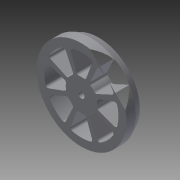
# Autodesk Inventor part: Colossus_7kW_Rotor
Saved by Autodesk Inventor 2014 (Build 180170000, 170)
## iProperties
Created: 2014-11-23
Part Number: Colossus_7kW_Rotor
Material: Générique
Document SubType Name: Modeling
Designer: Yann
Density: 1 g/cm^3
Appearance: Par défaut
Author: Yann
Autodesk Inventor part; units mm, degrees
ref_plane "YZ Plane" through (0, 0, 0) normal (1, 0, 0) x (0, 1, 0)
ref_plane "XZ Plane" through (0, 0, 0) normal (0, 1, 0) x (-1, 0, 0)
ref_plane "XY Plane" through (0, 0, 0) normal (0, 0, 1) x (1, 0, 0)
sketch "Esquisse1" plane through (0, 0, 0) normal (0, 1, 0) x (-1, 0, 0)
  arc A0 (26.7424, 50.7333) -> (-26.7424, 50.7333) centre (0, 0) ccw
  circle A1 centre (0, 0) radius 57.35
  line L0 (0, -80.29) -> (0, 80.29) construction
  line L1 (-80.29, 0) -> (80.29, 0) construction
  circle A2 centre (0, 0) radius 4
  line L2 (-6.2691, 21.7137) -> (-13.6461, 41.982)
  line L3 (13.6461, 41.982) -> (6.2691, 21.7137)
  arc A3 (11.5595, 45.9173) -> (-11.5595, 45.9173) centre (0, 0) ccw
  arc A4 (-11.5595, 45.9173) -> (-13.6461, 41.982) centre (-10.8271, 43.0081) ccw
  arc A5 (13.6461, 41.982) -> (11.5595, 45.9173) centre (10.8271, 43.0081) ccw
  circle A6 centre (0, 0) radius 16 construction
  circle A7 centre (0, 0) radius 57.35 construction
  arc A8 (3, 19.7737) -> (-3, 19.7737) centre (0, 0) ccw
  arc A9 (-6.2691, 21.7137) -> (-3, 19.7737) centre (-3.45, 22.7398) ccw
  arc A10 (3, 19.7737) -> (6.2691, 21.7137) centre (3.45, 22.7398) ccw
  line L4 (-19.7868, 10.921) -> (-39.3351, 20.0365)
  line L5 (-20.0365, 39.3351) -> (-10.921, 19.7868)
  arc A11 (-24.2947, 40.6422) -> (-40.6422, 24.2947) centre (0, 0) ccw
  arc A12 (-40.6422, 24.2947) -> (-39.3351, 20.0365) centre (-38.0672, 22.7554) ccw
  arc A13 (-20.0365, 39.3351) -> (-24.2947, 40.6422) centre (-22.7554, 38.0672) ccw
  arc A14 (-11.8608, 16.1035) -> (-16.1035, 11.8608) centre (0, 0) ccw
  arc A15 (-19.7868, 10.921) -> (-16.1035, 11.8608) centre (-18.519, 13.6399) ccw
  arc A16 (-11.8608, 16.1035) -> (-10.921, 19.7868) centre (-13.6399, 18.519) ccw
  line L6 (-21.7137, -6.2691) -> (-41.982, -13.6461)
  line L7 (-41.982, 13.6461) -> (-21.7137, 6.2691)
  arc A17 (-45.9173, 11.5595) -> (-45.9173, -11.5595) centre (0, 0) ccw
  arc A18 (-45.9173, -11.5595) -> (-41.982, -13.6461) centre (-43.0081, -10.8271) ccw
  arc A19 (-41.982, 13.6461) -> (-45.9173, 11.5595) centre (-43.0081, 10.8271) ccw
  arc A20 (-19.7737, 3) -> (-19.7737, -3) centre (0, 0) ccw
  arc A21 (-21.7137, -6.2691) -> (-19.7737, -3) centre (-22.7398, -3.45) ccw
  arc A22 (-19.7737, 3) -> (-21.7137, 6.2691) centre (-22.7398, 3.45) ccw
  line L8 (-10.921, -19.7868) -> (-20.0365, -39.3351)
  line L9 (-39.3351, -20.0365) -> (-19.7868, -10.921)
  arc A23 (-40.6422, -24.2947) -> (-24.2947, -40.6422) centre (0, 0) ccw
  arc A24 (-24.2947, -40.6422) -> (-20.0365, -39.3351) centre (-22.7554, -38.0672) ccw
  arc A25 (-39.3351, -20.0365) -> (-40.6422, -24.2947) centre (-38.0672, -22.7554) ccw
  arc A26 (-16.1035, -11.8608) -> (-11.8608, -16.1035) centre (0, 0) ccw
  arc A27 (-10.921, -19.7868) -> (-11.8608, -16.1035) centre (-13.6399, -18.519) ccw
  arc A28 (-16.1035, -11.8608) -> (-19.7868, -10.921) centre (-18.519, -13.6399) ccw
  line L10 (6.2691, -21.7137) -> (13.6461, -41.982)
  line L11 (-13.6461, -41.982) -> (-6.2691, -21.7137)
  arc A29 (-11.5595, -45.9173) -> (11.5595, -45.9173) centre (0, 0) ccw
  arc A30 (11.5595, -45.9173) -> (13.6461, -41.982) centre (10.8271, -43.0081) ccw
  arc A31 (-13.6461, -41.982) -> (-11.5595, -45.9173) centre (-10.8271, -43.0081) ccw
  arc A32 (-3, -19.7737) -> (3, -19.7737) centre (0, 0) ccw
  arc A33 (6.2691, -21.7137) -> (3, -19.7737) centre (3.45, -22.7398) ccw
  arc A34 (-3, -19.7737) -> (-6.2691, -21.7137) centre (-3.45, -22.7398) ccw
  line L12 (19.7868, -10.921) -> (39.3351, -20.0365)
  line L13 (20.0365, -39.3351) -> (10.921, -19.7868)
  arc A35 (24.2947, -40.6422) -> (40.6422, -24.2947) centre (0, 0) ccw
  arc A36 (40.6422, -24.2947) -> (39.3351, -20.0365) centre (38.0672, -22.7554) ccw
  arc A37 (20.0365, -39.3351) -> (24.2947, -40.6422) centre (22.7554, -38.0672) ccw
  arc A38 (11.8608, -16.1035) -> (16.1035, -11.8608) centre (0, 0) ccw
  arc A39 (19.7868, -10.921) -> (16.1035, -11.8608) centre (18.519, -13.6399) ccw
  arc A40 (11.8608, -16.1035) -> (10.921, -19.7868) centre (13.6399, -18.519) ccw
  line L14 (21.7137, 6.2691) -> (41.982, 13.6461)
  line L15 (41.982, -13.6461) -> (21.7137, -6.2691)
  arc A41 (45.9173, -11.5595) -> (45.9173, 11.5595) centre (0, 0) ccw
  arc A42 (45.9173, 11.5595) -> (41.982, 13.6461) centre (43.0081, 10.8271) ccw
  arc A43 (41.982, -13.6461) -> (45.9173, -11.5595) centre (43.0081, -10.8271) ccw
  arc A44 (19.7737, -3) -> (19.7737, 3) centre (0, 0) ccw
  arc A45 (21.7137, 6.2691) -> (19.7737, 3) centre (22.7398, 3.45) ccw
  arc A46 (19.7737, -3) -> (21.7137, -6.2691) centre (22.7398, -3.45) ccw
  line L16 (10.921, 19.7868) -> (20.0365, 39.3351)
  line L17 (39.3351, 20.0365) -> (19.7868, 10.921)
  arc A47 (40.6422, 24.2947) -> (24.2947, 40.6422) centre (0, 0) ccw
  arc A48 (24.2947, 40.6422) -> (20.0365, 39.3351) centre (22.7554, 38.0672) ccw
  arc A49 (39.3351, 20.0365) -> (40.6422, 24.2947) centre (38.0672, 22.7554) ccw
  arc A50 (16.1035, 11.8608) -> (11.8608, 16.1035) centre (0, 0) ccw
  arc A51 (10.921, 19.7868) -> (11.8608, 16.1035) centre (13.6399, 18.519) ccw
  arc A52 (16.1035, 11.8608) -> (19.7868, 10.921) centre (18.519, 13.6399) ccw
  point P0 (0, 0)
  point P1 (-14.7432, 44.9962)
  point P2 (14.7432, 44.9962)
  point P3 (5.3773, 19.2636)
  point P4 (-5.3773, 19.2636)
  point P5 (-42.2422, 21.3921)
  point P6 (-21.3921, 42.2422)
  point P7 (-9.8191, 17.4237)
  point P8 (-17.4237, 9.8191)
  point P9 (-44.9962, -14.7432)
  point P10 (-44.9962, 14.7432)
  point P11 (-19.2636, 5.3773)
  point P12 (-19.2636, -5.3773)
  point P13 (-21.3921, -42.2422)
  point P14 (-42.2422, -21.3921)
  point P15 (-17.4237, -9.8191)
  point P16 (-9.8191, -17.4237)
  point P17 (14.7432, -44.9962)
  point P18 (-14.7432, -44.9962)
  point P19 (-5.3773, -19.2636)
  point P20 (5.3773, -19.2636)
  point P21 (42.2422, -21.3921)
  point P22 (21.3921, -42.2422)
  point P23 (9.8191, -17.4237)
  point P24 (17.4237, -9.8191)
  point P25 (44.9962, 14.7432)
  point P26 (44.9962, -14.7432)
  point P27 (19.2636, -5.3773)
  point P28 (19.2636, 5.3773)
  point P29 (21.3921, 42.2422)
  point P30 (42.2422, 21.3921)
  point P31 (17.4237, 9.8191)
  point P32 (9.8191, 17.4237)
  dimension "d0" = 8
  dimension "d2" = 3
  dimension "d3" = 10
  dimension "d5" = 40
  dimension "d15" = 20
  dimension "d16" = 3
  dimension "d17" = 6
  dimension "d20" = 360
  constraints: 130 point on circle, 51 centre point, 32 end point, 32 point on line, 9 tangent, 5 coincident, 3 equal radius, 1 symmetric about line, 210 other
  measures "d0" diameter of A2
  measures "d2" radius of A4
  measures "d3" radial gap between concentric circles of A3 A1
  measures "d5" angle of L3 L2
  measures "d15" radius of A8
  measures "d16" radius of A9
  measures "d17" distance of A8.start A8.end
extrude "Extrusion1" add sketch "Esquisse1" against normal blind 22
chamfer "Chanfrein1" distance 18 angle 25 1 edges at (57.35, 0, 0) measured on face at (57.35, -0.5, 0)
